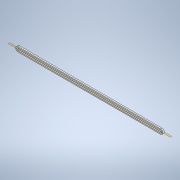
# Autodesk Inventor part: 零件4
Saved by Autodesk Inventor 2022 (Build 260153000, 153)
## iProperties
Created: 2023-04-16
Part Number: 零件4
Material: 一般
Document SubType Name: Modeling
Designer: JOU
Density: 1 g/cm^3
Appearance: 預設
Author: JOU
Autodesk Inventor part; units mm, degrees
ref_plane "YZ Plane" through (0, 0, 0) normal (1, 0, 0) x (0, 1, 0)
ref_plane "XZ Plane" through (0, 0, 0) normal (0, 1, 0) x (-1, 0, 0)
ref_plane "XY Plane" through (0, 0, 0) normal (0, 0, 1) x (1, 0, 0)
sketch "草圖1" plane through (0, 0, 0) normal (0, 0, 1) x (1, 0, 0)
  line L0 (0, 0) -> (300, 0) construction
  line L1 (0, -5) -> (300, -5)
  line L2 (300, 5) -> (0, 5)
  arc A0 (0, 5) -> (0, -5) centre (0, 0) ccw
  arc A1 (300, -5) -> (300, 5) centre (300, 0) ccw
  line L3 (0, 0) -> (300, 0) construction
  line L4 (0, -2.5) -> (300, -2.5)
  line L5 (300, 2.5) -> (0, 2.5)
  arc A2 (0, 2.5) -> (0, -2.5) centre (0, 0) ccw
  arc A3 (300, -2.5) -> (300, 2.5) centre (300, 0) ccw
  point P0 (150, 0)
  point P1 (150, 0)
  dimension "d0" = 5
  dimension "d1" = 10
  dimension "d2" = 300
  constraints: 16 end point, 8 point on circle, 8 tangent, 4 centre point, 3 equal length, 2 midpoint, 1 coincident, 1 horizontal
  measures "d0" distance between parallel lines of L4 L5
  measures "d1" distance between parallel lines of L1 L2
  measures "d2" distance of L2.start L2.end
extrude "擠出1" add sketch "草圖1" along normal blind 3
ref_plane "工作平面1" through (0, 0, 0) normal (0, 1, 0) x (1, 0, 0)
